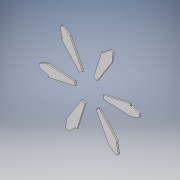
# Autodesk Inventor part: SpurGear
Saved by Autodesk Inventor 2019.3 (Build 233278000, 278)
## iProperties
Created: 2019-09-04
Part Number: SpurGear
Material: Generic
Document SubType Name: Modeling
Designer: Frienddo
Density: 1 g/cm^3
Appearance: Default
Author: Frienddo
Autodesk Inventor part; units mm, degrees
ref_plane "YZ Plane" through (0, 0, 0) normal (1, 0, 0) x (0, 1, 0)
ref_plane "XZ Plane" through (0, 0, 0) normal (0, 1, 0) x (-1, 0, 0)
ref_plane "XY Plane" through (0, 0, 0) normal (0, 0, 1) x (1, 0, 0)
sketch "Base" plane through (0, 0, 0) normal (0, 0, 1) x (1, 0, 0)
  circle A0 centre (0, 0) radius 215 construction
  circle A1 centre (0, 0) radius 217.5139 construction
  circle A2 centre (0, 0) radius 240 construction
  circle A3 centre (0, 0) radius 260 construction
  line L0 (197.1345, 91.9253) -> (240, 0) construction
  line L1 (-364.0417, 0) -> (364.2503, 0) construction
  line L2 (197.1345, 91.9253) -> (0, 0) construction
  line L3 (240, 0) -> (82.7311, -73.3357) construction
  arc A4 (217.3109, -9.3953) -> (259.7995, 10.2076) centre (121.323, 254.5037) ccw
  line L4 (259.7995, 10.2076) -> (258.9093, 23.7904)
  arc A5 (258.9093, 23.7904) -> (214.2254, 37.6797) centre (153.5044, -236.4905) ccw
  line L5 (214.2254, 37.6797) -> (211.7495, 37.2442)
  line L6 (209.8838, 46.6239) -> (0, 0)
  line L7 (217.3109, -9.3953) -> (0, 0)
  line L8 (237.9468, 31.3263) -> (0, 0) construction
  line L9 (259.3544, 16.999) -> (0, 0) construction
  line L10 (258.9093, 23.7904) -> (0, 0) construction
  line L11 (259.7995, 10.2076) -> (0, 0) construction
  line L12 (219.1565, 14.2535) -> (213.024, 43.9664) construction
  line L13 (219.1565, 14.2535) -> (189.1909, 9.5074) construction
  line L14 (210.876, 67.8334) -> (214.2254, 37.6797) construction
  line L15 (210.876, 67.8334) -> (180.9103, 63.0873) construction
  circle A6 centre (0, 0) radius 75
  line L16 (0, -364) -> (0, 364) construction
  line L17 (20, 47.2842) -> (-20, 47.2842)
  line L18 (-20, 47.2842) -> (-20, 87.2842)
  line L19 (-20, 87.2842) -> (20, 87.2842)
  line L20 (20, 87.2842) -> (20, 47.2842)
  line L21 (20, 47.2842) -> (-20, 87.2842) construction
  line L22 (-20, 47.2842) -> (20, 87.2842) construction
  line L23 (-20, 72.2842) -> (20, 72.2842) construction
  line L24 (209.8838, 46.6239) -> (211.7495, 37.2442)
  point P0 (0, 67.2842)
  dimension "sdTemp" = 8
  dimension "RefDiam" = 24
  dimension "RootDiam" = 14
  dimension "BaseDiam" = 23.9087
  dimension "TipDiam" = 32
  dimension "Pitch" = 60
  dimension "ToothThick" = 30
  dimension "InnerToothThick" = 12
  dimension "kwdTemp" = 11
  dimension "kwTemp" = 9
  dimension "khTemp" = 10
  constraints: 46 end point, 16 point on circle, 6 centre point, 6 coincident, 4 perpendicular, 4 point on line, 3 midpoint, 2 parallel, 2 tangent, 1 horizontal, 5 other
extrude "GearOneTooth" add sketch "Base" along normal mid plane 7 contours L7 A6 L6 L24 L5 A5 L4 A4 | L7 L6 A6
pattern_circular "GearCircularPattern" count 6 over 360 about axis through (0, 0, -10) along (0, 0, 1) of "GearOneTooth"
extrude "Shaft" cut sketch "Base" along normal mid plane 7 contours A6 L18 L17 L20 L6 L7 | L7 L6 A6 | L18 L19 L20 A6 | A6 L20 L17 L18
equation "\"RootDiam\" = RefDiam - 2.5 * Module"
equation "\"TipDiam\" = RefDiam + 2 * Module"
equation "\"ToothThick\" = 0.5 * Pitch"
equation "\"InnerToothThick\" = 0.2 * Pitch"
equation "\"Module\" = 4"
equation "\"ReferencePressureAngle\" = 5deg"
equation "\"Thickness\" = 7"
equation "\"ShaftDiameter\" = 8"
equation "\"KeyWidth\" = 9"
equation "\"KeywayDepth\" = 11"
body "Solid1"
